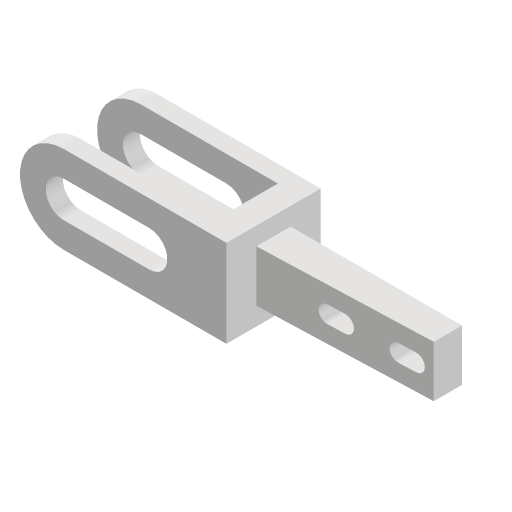
# Autodesk Inventor part: fan_holder_0301
Saved by Autodesk Inventor 2024 (Build 280153000, 153)
## iProperties
Created: 2023-02-14
Part Number: fan_holder_0301
Material: 一般
Document SubType Name: Modeling
Designer: USER
Density: 1 g/cm^3
Appearance: 預設
Author: USER
Autodesk Inventor part; units mm, degrees
ref_plane "YZ Plane" through (0, 0, 0) normal (1, 0, 0) x (0, 1, 0)
ref_plane "XZ Plane" through (0, 0, 0) normal (0, 1, 0) x (-1, 0, 0)
ref_plane "XY Plane" through (0, 0, 0) normal (0, 0, 1) x (1, 0, 0)
sketch "草圖17" plane through (0, 0, 0) normal (0, 0, 1) x (1, 0, 0)
  line L0 (-12.5, -3) -> (12.5, -3)
  line L1 (12.5, -3) -> (12.5, 3)
  line L2 (12.5, 3) -> (-12.5, 3)
  line L3 (-12.5, 3) -> (-12.5, -3)
  line L4 (-12.5, -3) -> (12.5, 3) construction
  line L5 (12.5, -3) -> (-12.5, 3) construction
  line L6 (0, 0) -> (-6.6625, 0) construction
  circle A0 centre (9.5, 0) radius 2
  line L7 (-2.5, 0) -> (-4.5, 0) construction
  line L8 (-2.5, 1) -> (-4.5, 1)
  line L9 (-4.5, -1) -> (-2.5, -1)
  arc A1 (-2.5, -1) -> (-2.5, 1) centre (-2.5, 0) ccw
  arc A2 (-4.5, 1) -> (-4.5, -1) centre (-4.5, 0) ccw
  line L10 (5.5, -0.0384) -> (3.5, -0.0384) construction
  line L11 (5.5, 0.9616) -> (3.5, 0.9616)
  line L12 (3.5, -1.0384) -> (5.5, -1.0384)
  arc A3 (5.5, -1.0384) -> (5.5, 0.9616) centre (5.5, -0.0384) ccw
  arc A4 (3.5, 0.9616) -> (3.5, -1.0384) centre (3.5, -0.0384) ccw
  line L13 (7.5, 3) -> (7.5, -3)
  point P0 (-3.5, 0)
  point P1 (4.5, -0.0384)
  dimension "d166" = 25
  dimension "d167" = 6
  dimension "d170" = 4
  dimension "d171" = 3
  dimension "d173" = 2
  dimension "d174" = 12
  dimension "d175" = 2
  dimension "d190" = 4
  dimension "d191" = 2
  dimension "d192" = 2
  constraints: 32 end point, 8 point on circle, 8 tangent, 5 centre point, 5 point on line, 4 midpoint, 4 parallel, 3 horizontal, 2 perpendicular, 1 equal radius
  measures "d166" distance of L1.end L2.end
  measures "d167" distance of L0.end L1.end
  measures "d170" diameter of A0
  measures "d171" distance from line of L1 A0.centre
  measures "d173" diameter of A2
  measures "d174" distance of A0.centre L7.start
  measures "d175" distance of L7.end L7.start
  measures "d190" horizontal distance of L10.start A0.centre
  measures "d191" distance of L10.end L10.start
  measures "d192" distance from line of L10.start L13
extrude "擠出18" add sketch "草圖17" along normal mid plane 4 contours L3 L2 L13 L0
sketch "草圖18" plane through (0, 0, 0) normal (0, 0, 1) x (1, 0, 0)
  line L0 (7.5, -3) -> (-12.5, -3) projected
  line L1 (-12.5, -3) -> (-12.5, 3) projected
  line L2 (-12.5, 3) -> (7.5, 3) projected
  arc A0 (-2.5, -1) -> (-2.5, 1) centre (-2.5, 0) ccw projected
  line L3 (-2.5, 1) -> (-4.5, 1) projected
  arc A1 (-4.5, 1) -> (-4.5, -1) centre (-4.5, 0) ccw projected
  line L4 (-4.5, -1) -> (-2.5, -1) projected
  line L5 (-12.5, -5.1) -> (-21.5, -5.1)
  line L6 (-21.5, -5.1) -> (-21.5, 5.1)
  line L7 (-21.5, 5.1) -> (-12.5, 5.1)
  line L8 (-12.5, 5.1) -> (-12.5, -5.1)
  line L9 (-12.5, -5.1) -> (-21.5, 5.1) construction
  line L10 (-21.5, -5.1) -> (-12.5, 5.1) construction
  arc A2 (-2.5, -1) -> (-2.5, 1) centre (-2.5, 0) ccw construction
  line L11 (-2.5, 0) -> (-4.5, 0) construction
  line L12 (-21.5, 0) -> (-31.5, 0) construction
  line L13 (-21.5, 2.1) -> (-31.5, 2.1)
  line L14 (-31.5, -2.1) -> (-21.5, -2.1)
  arc A3 (-21.5, -2.1) -> (-21.5, 2.1) centre (-21.5, 0) ccw
  arc A4 (-31.5, 2.1) -> (-31.5, -2.1) centre (-31.5, 0) ccw
  line L15 (-31.5, 5.1) -> (-21.5, 5.1)
  arc A5 (-21.5, -5.1) -> (-21.5, 5.1) centre (-21.5, 0) ccw
  line L16 (-21.5, -5.1) -> (-31.5, -5.1)
  arc A6 (-31.5, 5.1) -> (-31.5, -5.1) centre (-31.5, 0) ccw
  line L17 (-12.5, -3) -> (-12.5, 3) construction
  line L18 (7.5, 3) -> (7.5, -3) projected
  point P0 (0, 0)
  point P1 (-17, 0)
  point P2 (-26.5, 0)
  dimension "d181" = 2.1
  dimension "d182" = 10
  dimension "d183" = 3
  dimension "d189" = 9
  constraints: 26 end point, 8 point on circle, 4 centre point, 4 midpoint, 4 parallel, 4 tangent, 3 horizontal, 2 collinear, 2 point on line, 1 perpendicular, 3 other
  measures "d181" radius of A3
  measures "d182" distance of L12.end L12.start
  measures "d183" distance between parallel lines of L13 L15
  measures "d189" distance from line of L8 L12.start
extrude "擠出19" add sketch "草圖18" along normal mid plane 11 contours L8 L5 A5 L7 L1 | L16 A6 L15 L6 L13 A4 L14 | L6 A3 A5
sketch "草圖19" plane through (0, 0, 0) normal (0, 0, 1) x (1, 0, 0)
  arc A0 (-31.5, 5.1) -> (-31.5, -5.1) centre (-31.5, 0) ccw projected
  line L0 (-31.5, 5.1) -> (-12.5, 5.1) projected
  line L1 (-12.5, 5.1) -> (-12.5, -5.1) projected
  line L2 (-12.5, -5.1) -> (-31.5, -5.1) projected
  arc A1 (-21.5, -2.1) -> (-21.5, 2.1) centre (-21.5, 0) ccw projected
  line L3 (-21.5, 2.1) -> (-31.5, 2.1) projected
  arc A2 (-31.5, 2.1) -> (-31.5, -2.1) centre (-31.5, 0) ccw projected
  line L4 (-31.5, -2.1) -> (-21.5, -2.1) projected
  line L5 (-15.5, -5.1) -> (-45.605, -5.1)
  line L6 (-45.605, -5.1) -> (-45.605, 5.1)
  line L7 (-45.605, 5.1) -> (-15.5, 5.1)
  line L8 (-15.5, 5.1) -> (-15.5, -5.1)
  line L9 (-31.5, 5.1) -> (-12.5, 5.1) projected
  point P0 (0, 0)
  point P1 (-15.5, 5.1)
  dimension "d186" = 3
  constraints: 8 end point, 2 parallel, 1 collinear, 1 horizontal, 1 perpendicular, 1 point on line
  measures "d186" distance between parallel lines of L1 L8
extrude "擠出20" cut sketch "草圖19" along normal mid plane 7 contours L0 L8 L2 A0 | A0 L5 L6 L7
sketch "草圖20" plane through (7.5, 3, 2) normal (0, 1, 0) x (1, 0, 0)
  line L0 (0, 0) -> (-20, 0) projected
  line L1 (-20, 0) -> (0, 0.6984)
  line L2 (0, 4) -> (0, 0) projected
  point P0 (-7.5, 2)
  dimension "d193" = 20
  dimension "d194" = 2
  constraints: 2 end point, 2 point on line
  measures "d193" distance of L0.start point (-20, 0)
  measures "d194" angle of L0 L1
extrude "擠出21" cut sketch "草圖20" against normal through all
